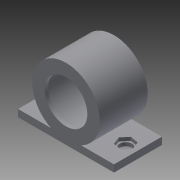
# Autodesk Inventor part: bart xl rjmp 2 part bearing holder v6
Saved by Autodesk Inventor 2014 SP1 (Build 180222100, 222)
## iProperties
Created: 2015-09-03
Part Number: bart xl rjmp 2 part bearing holder v6
Material: Generic
Document SubType Name: Modeling
Designer: dave
Density: 1 g/cm^3
Appearance: Default
Author: dave
Autodesk Inventor part; units mm, degrees
ref_plane "YZ Plane" through (0, 0, 0) normal (1, 0, 0) x (0, 1, 0)
ref_plane "XZ Plane" through (0, 0, 0) normal (0, 1, 0) x (-1, 0, 0)
ref_plane "XY Plane" through (0, 0, 0) normal (0, 0, 1) x (1, 0, 0)
sketch "Sketch1" plane through (0, 0, 0) normal (0, 0, 1) x (1, 0, 0)
  line L0 (0, 0) -> (27, 0)
  line L1 (27, 0) -> (27, 13.5)
  line L2 (27, 13.5) -> (0, 13.5)
  line L3 (0, 13.5) -> (0, 0)
  line L4 (13.4862, 18.9079) -> (13.4862, -5.216) construction
  line L5 (13.4862, -5.216) -> (23.4862, -5.216) construction
  line L6 (23.4862, -5.216) -> (23.4862, 20) construction
  line L7 (23.4862, 20) -> (3.4862, 20) construction
  line L8 (3.4862, 20) -> (3.4862, -7.3205) construction
  line L9 (14, 12) -> (14, 9) construction
  line L10 (13.5, 13.5) -> (13.5, 8.6504) construction
  line L11 (13.5, 8.6504) -> (13.5, 6.3397) construction
  line L12 (-7, 6.846) -> (36, 6.846) construction
  point P0 (3.4862, 6.846)
  point P1 (23.4862, 6.846)
  dimension "d0" = 27
  dimension "d1" = 13.5
  dimension "d2" = 10
  dimension "d3" = 20
  constraints: 26 end point, 6 parallel, 5 point on line, 4 perpendicular, 1 horizontal, 1 midpoint
  measures "d0" distance of L2.end L1.end
  measures "d1" distance of L1.end L0.end
  measures "d2" distance of L4.end L5.end
  measures "d3" distance of L6.end L7.end
extrude "Extrusion1" add sketch "Sketch1" along normal blind 2
hole "Hole1" at (3.4862, 6.846, 0) at (23.4862, 6.846, 0) direction (0, 0, 1) diameter 3.5 end through all
sketch "Sketch2" plane through (0, 0, 2) normal (0, 0, 1) x (1, 0, 0)
  circle A0 centre (3.4862, 6.846) radius 1.75 projected
  circle A1 centre (23.4862, 6.846) radius 1.75 projected
  line L0 (5, 5) -> (2.6444, 4.6119)
  line L1 (2.6444, 4.6119) -> (1.1306, 6.4579)
  line L2 (1.1306, 6.4579) -> (1.9723, 8.6919)
  line L3 (1.9723, 8.6919) -> (4.3279, 9.08)
  line L4 (4.3279, 9.08) -> (5.8417, 7.234)
  line L5 (5.8417, 7.234) -> (5, 5)
  line L6 (24.3353, 4.6119) -> (21.976, 4.9936)
  line L7 (21.976, 4.9936) -> (21.1269, 7.2276)
  line L8 (21.1269, 7.2276) -> (22.637, 9.08)
  line L9 (22.637, 9.08) -> (24.9963, 8.6983)
  line L10 (24.9963, 8.6983) -> (25.8454, 6.4643)
  line L11 (25.8454, 6.4643) -> (24.3353, 4.6119)
  constraints: 24 end point, 2 coincident, 26 other
extrude "Extrusion2" cut sketch "Sketch2" against normal blind 1 contours L0 L1 L2 L3 L4 L5
extrude "Extrusion3" cut sketch "Sketch2" against normal blind 1 contours L6 L7 L8 L9 L10 L11
sketch "Sketch4" plane through (0, 0, 0) normal (0, 1, 0) x (-1, 0, 0)
  line L0 (-6.7373, -10.6634) -> (-6.7373, -4.6634) construction
  line L1 (-27, -7.5) -> (0, -7.5) construction
  line L2 (0, -7.5) -> (-27, -7.5) construction
  line L3 (-13.5, -7.5) -> (-13.5, 2) construction
  arc A0 (-9.2574, 2) -> (-17.7426, 2) centre (-13.5, 10.5) ccw
  circle A1 centre (-13.5, 10.5) radius 8.25
  line L4 (-9.2574, 2) -> (-17.7426, 2)
  point P0 (0, 0)
  dimension "d17" = 9.5
  dimension "d18" = 19
  dimension "d19" = 16.5
  constraints: 10 end point, 3 perpendicular, 2 centre point, 2 point on circle, 1 coincident, 1 collinear, 1 midpoint
  measures "d17" distance of L3.end L3.start
  measures "d18" diameter of A0
  measures "d19" diameter of A1
extrude "Extrusion4" add sketch "Sketch4" along normal blind 13.5
sketch "Sketch5" plane through (0, 0, 0) normal (0, -1, 0) x (1, 0, 0)
  circle A0 centre (13.5, 10.5) radius 8.25 projected
  circle A1 centre (13.5, 10.5) radius 6
  circle A2 centre (13.5, 10.5) radius 8.25
  dimension "d22" = 12
  constraints: 2 centre point, 2 coincident, 1 concentric
  measures "d22" diameter of A1
extrude "Extrusion5" add sketch "Sketch5" against normal blind 1
body "Solid1"
